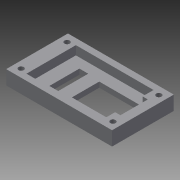
# Autodesk Inventor part: suport releu
Saved by Autodesk Inventor 2015 SP1 (Build 190203100, 203)
## iProperties
Created: 2015-08-09
Part Number: suport releu
Material: Generic
Document SubType Name: Modeling
Designer: ubik
Density: 1 g/cm^3
Appearance: Default
Author: ubik
Autodesk Inventor part; units mm, degrees
ref_plane "YZ Plane" through (0, 0, 0) normal (1, 0, 0) x (0, 1, 0)
ref_plane "XZ Plane" through (0, 0, 0) normal (0, 1, 0) x (-1, 0, 0)
ref_plane "XY Plane" through (0, 0, 0) normal (0, 0, 1) x (1, 0, 0)
sketch "Sketch1" plane through (0, 0, 0) normal (0, 0, 1) x (1, 0, 0)
  line L0 (-30, 17.5) -> (30, 17.5)
  line L1 (30, 17.5) -> (30, -17.5)
  line L2 (30, -17.5) -> (-30, -17.5)
  line L3 (-30, -17.5) -> (-30, 17.5)
  line L4 (-2.5, 7.75) -> (25, 7.75)
  line L5 (25, 7.75) -> (25, -7.75)
  line L6 (25, -7.75) -> (-2.5, -7.75)
  line L7 (-2.5, -7.75) -> (-2.5, 7.75)
  line L8 (-14.5, 8.5) -> (-9.5, 8.5)
  line L9 (-9.5, 8.5) -> (-9.5, -8.5)
  line L10 (-9.5, -8.5) -> (-14.5, -8.5)
  line L11 (-14.5, -8.5) -> (-14.5, 8.5)
  point P0 (0, 0)
  dimension "length" = 60
  dimension "width" = 35
  dimension "d2" = 17.5
  dimension "d3" = 30
  dimension "d4" = 27.5
  dimension "d5" = 15.5
  dimension "d6" = 7.75
  dimension "d7" = 5
  dimension "d8" = 5
  dimension "d9" = 17
  dimension "d10" = 8.5
  dimension "d11" = 7
  constraints: 24 end point, 6 parallel, 3 horizontal, 3 perpendicular
  measures "length" distance of L1.end L2.end
  measures "width" distance of L0.end L1.end
  measures "d2" distance from line of point (0, 0) L0
  measures "d3" distance from line of point (0, 0) L3
  measures "d4" distance of L4.start L4.end
  measures "d5" distance of L6.end L4.start
  measures "d6" distance from line of point (0, 0) L4
  measures "d7" distance between parallel lines of L1 L5
  measures "d8" distance of L8.start L8.end
  measures "d9" distance of L10.end L8.start
  measures "d10" distance from line of point (0, 0) L8
  measures "d11" distance between parallel lines of L7 L9
extrude "Extrusion1" add sketch "Sketch1" along normal blind 3
sketch "Sketch2" plane through (0, 0, 3) normal (0, 0, 1) x (1, 0, 0)
  line L0 (-22, 9) -> (22, 9)
  line L1 (22, 9) -> (22, -9)
  line L2 (22, -9) -> (-22, -9)
  line L3 (-22, -9) -> (-22, 9)
  line L4 (25, 7.75) -> (25, -7.75) projected
  line L5 (25, -7.75) -> (-2.5, -7.75) projected
  line L6 (-2.5, -7.75) -> (-2.5, 7.75) projected
  line L7 (-2.5, 7.75) -> (25, 7.75) projected
  line L8 (-9.5, 8.5) -> (-9.5, -8.5) projected
  line L9 (-9.5, -8.5) -> (-14.5, -8.5) projected
  line L10 (-14.5, -8.5) -> (-14.5, 8.5) projected
  line L11 (-14.5, 8.5) -> (-9.5, 8.5) projected
  line L12 (30, 17.5) -> (-30, 17.5) projected
  line L13 (-30, 17.5) -> (-30, -17.5) projected
  line L14 (-30, -17.5) -> (30, -17.5) projected
  line L15 (30, -17.5) -> (30, 17.5) projected
  point P0 (0, 0)
  dimension "d14" = 44
  dimension "d15" = 18
  dimension "d16" = 9
  constraints: 8 end point, 2 parallel, 1 horizontal, 1 perpendicular
  measures "d14" distance of L0.start L0.end
  measures "d15" distance of L2.end L0.start
  measures "d16" distance from line of point (0, 0) L0
extrude "Extrusion2" add sketch "Sketch2" along normal blind 5 contours L7 L4 L5 L1 | L15 L14 L13 L12
hole "Hole1" at (-26, 13, 0) direction (0, 0, 1) diameter 3 end through all
pattern_linear "Rectangular Pattern1" count 2 spacing 52 along (1, 0, 0) count 2 spacing 26 along (0, -1, 0) of "Hole1"
sketch "Sketch3" plane through (0, 0, 3) normal (0, 0, -1) x (-1, 0, 0)
  line L0 (-25, -7.75) -> (-22, -7.75) projected
  line L1 (-22, -7.75) -> (-22, 7.75) projected
  line L2 (-22, 7.75) -> (-25, 7.75) projected
  line L3 (-25, 7.75) -> (-25, -7.75) projected
  point P0 (0, 0)
extrude "Extrusion3" cut sketch "Sketch3" against normal through all
sketch "Sketch4" plane through (-22, 9, 3) normal (0, -1, 0) x (1, 0, 0)
  line L0 (44, 0) -> (0, 0) projected
  line L1 (44, 0) -> (44, 5) projected
  line L2 (0, 5) -> (44, 5) projected
  line L3 (0, 0) -> (0, 5) projected
  point P0 (22, -3)
extrude "Extrusion4" cut sketch "Sketch4" against normal blind 5
sketch "Sketch5" plane through (-22, -9, 3) normal (0, 1, 0) x (1, 0, 0)
  line L0 (0, 0) -> (44, 0) projected
  line L1 (0, 0) -> (0, -5) projected
  line L2 (44, -5) -> (0, -5) projected
  line L3 (44, 0) -> (44, -5) projected
  point P0 (22, 3)
extrude "Extrusion5" cut sketch "Sketch5" against normal blind 5
equation "\"d2\" = 0.5 * width"
equation "\"d3\" = 0.5 * length"
equation "\"d6\" = 0.5 * d5"
equation "\"d10\" = 0.5 * d9"
equation "\"d16\" = 0.5 * d15"
body "Solid1"
